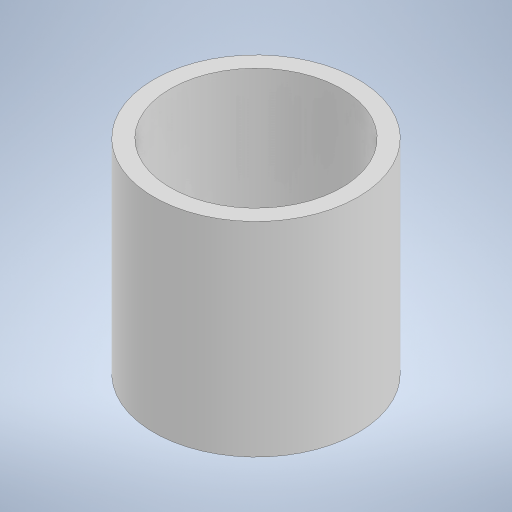
# Autodesk Inventor part: втулка_5-4
Saved by Autodesk Inventor 2024 (Build 280153000, 153)
## iProperties
Created: 2026-08-01
Part Number: втулка_5-4
Material: Типовые
Document SubType Name: Modeling
Designer: ejenie
Density: 1 g/cm^3
Appearance: По умолчанию
Author: ejenie
Autodesk Inventor part; units mm, degrees
ref_plane "YZ Plane" through (0, 0, 0) normal (1, 0, 0) x (0, 1, 0)
ref_plane "XZ Plane" through (0, 0, 0) normal (0, 1, 0) x (-1, 0, 0)
ref_plane "XY Plane" through (0, 0, 0) normal (0, 0, 1) x (1, 0, 0)
sketch "Эскиз1" plane through (0, 0, 0) normal (0, 1, 0) x (-1, 0, 0)
  circle A0 centre (0, 0) radius 2.5
  circle A1 centre (0, 0) radius 2.1
  dimension "d0" = 5
  dimension "d1" = 4.2
  constraints: 2 centre point, 2 coincident
  measures "d0" diameter of A0
  measures "d1" diameter of A1
extrude "Выдавливание1" add sketch "Эскиз1" along normal blind 5
